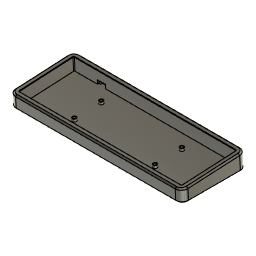
Quark MFR2 (Autodesk Fusion 360 design; units mm, degrees)
Autodesk Fusion 360 part; units mm, degrees
sketch "Sketch1" plane through (0, 0, 0) normal (0, 0, 1) x (1, 0, 0)
  line L0 (0, 0) -> (228.6, 0) construction
  line L1 (228.6, 0) -> (228.6, 76.2) construction
  line L2 (228.6, 76.2) -> (0, 76.2) construction
  line L3 (0, 76.2) -> (0, 0) construction
  line L4 (-0.5, -0.5) -> (229.1, -0.5)
  line L5 (229.1, -0.5) -> (229.1, 76.7)
  line L6 (229.1, 76.7) -> (-0.5, 76.7)
  line L7 (-0.5, 76.7) -> (-0.5, -0.5)
  line L8 (-7.5, 83.7) -> (-7.5, -7.5)
  line L9 (-7.5, -7.5) -> (236.1, -7.5)
  line L10 (236.1, -7.5) -> (236.1, 83.7)
  line L11 (236.1, 83.7) -> (-7.5, 83.7)
  dimension "d1" = 228.6
  dimension "d2" = 76.2
  dimension "d3" = 0.5
  dimension "d4" = 7.5
  constraint horizontal L0
  constraint vertical L1
  constraint horizontal L2
  constraint vertical L3
  constraint coincident L0.start L3.end
  measures "d1" distance of L0.start L0.end
  measures "d2" distance of L0.start L2.end
ref_plane "WorkPlane1" through (114.3, 38.1, -3.46) normal (0, 0, 1) x (1, 0, 0)
ref_plane "WorkPlane2" through (114.3, 38.1, 14.6) normal (0, 0, 1) x (1, 0, 0)
extrude "Extrude1" add sketch "Sketch1" along normal up to surface (14.6 mm away) and the other way up to surface (3.46 mm away)
sketch "Sketch3" plane through (236.1, 0, 0) normal (1, 0, 0) x (0, 1, 0)
  line L0 (83.7, 14.6) -> (-7.5, 14.6)
  line L1 (-7.5, 14.6) -> (-7.5, -3.46)
  line L2 (-7.5, -3.46) -> (83.7, -3.46)
  line L3 (83.7, -3.46) -> (83.7, 14.6)
  line L4 (-7.5, 14.6) -> (-7.5, -3.6755)
  line L5 (-7.5, -3.6755) -> (92.363, -8.9091)
  line L6 (-7.5, -3.6755) -> (92.5, -3.6755) construction
  dimension "d11" = 18.2755
  dimension "d12" = 100
  dimension "d13" = 3
  constraint coincident L0.end L1.start
  constraint perpendicular L0 L4
  constraint horizontal L6
  measures "d11" distance of L0.end L4.end
  measures "d12" distance of L4.end L5.end
  measures "d13" angle of L5 L6
ref_plane "WorkPlane3" through (236.1, 42.4315, -6.2923) normal (0, -0.052336, -0.99863) x (0, 0.99863, -0.052336)
sketch "Sketch5" plane through (0, 0, -3.46) normal (0, 0, -1) x (1, 0, 0)
  line L0 (229.1, -76.7) -> (-0.5, -76.7)
  line L1 (-0.5, -76.7) -> (-0.5, 0.5)
  line L2 (-0.5, 0.5) -> (229.1, 0.5)
  line L3 (229.1, 0.5) -> (229.1, -76.7)
  line L4 (-7.5, 7.5) -> (-7.5, -83.7)
  line L5 (-7.5, -83.7) -> (236.1, -83.7)
  line L6 (236.1, -83.7) -> (236.1, 7.5)
  line L7 (236.1, 7.5) -> (-7.5, 7.5)
  line L8 (-7.5, 7.5) -> (236.1, 7.5)
  line L9 (236.1, 7.5) -> (236.1, -83.7)
  line L10 (236.1, -83.7) -> (-7.5, -83.7)
  line L11 (-7.5, -83.7) -> (-7.5, 7.5)
  constraint horizontal L8
  constraint vertical L9
  constraint horizontal L10
  constraint vertical L11
  constraint coincident L5.end L6.start
  constraint coincident L4.start L7.end
extrude "Extrude2" add sketch "Sketch5" along normal up to surface contours L0 L1 L2 L3 | L4 L5 L6 L7 L8 L9 L10 L11 end surface through (236.1, 42.4315, -6.2923) normal (0, -0.052336, -0.99863) offset 0
fillet "Fillet1" radius 9 1 edges at (236.1, -7.5, 5.4623)
fillet "Fillet2" radius 9 1 edges at (236.1, 83.7, 3.0725)
fillet "Fillet3" radius 9 1 edges at (-7.5, 83.7, 3.0725)
fillet "Fillet4" radius 9 1 edges at (-7.5, -7.5, 5.4623)
fillet "Fillet5" radius 1 1 edges at (229.1, 76.7, 5.57)
fillet "Fillet6" radius 1 1 edges at (-0.5, 76.7, 5.57)
fillet "Fillet7" radius 1 1 edges at (229.1, -0.5, 5.57)
fillet "Fillet8" radius 1 1 edges at (-0.5, -0.5, 5.57)
chamfer "Chamfer1" distance 2 angle 45 8 edges at (-7.5, 38.1, 14.6) (-4.864, 81.064, 14.6) (114.3, 83.7, 14.6) (233.464, 81.064, 14.6) (236.1, 38.1, 14.6) (233.464, -4.864, 14.6) (114.3, -7.5, 14.6) (-4.864, -4.864, 14.6)
chamfer "Chamfer2" distance 2 angle 45 8 edges at (-7.5, 38.1, -6.0653) (-4.864, -4.864, -3.8136) (114.3, -7.5, -3.6755) (233.464, -4.864, -3.8136) (236.1, 38.1, -6.0653) (233.464, 81.064, -8.3169) (114.3, 83.7, -8.4551) (-4.864, 81.064, -8.3169)
chamfer "Chamfer3" distance 0.5 angle 45 4 edges at (114.3, 76.7, 14.6) (-0.5, 38.1, 14.6) (114.3, -0.5, 14.6) (229.1, 38.1, 14.6)
extrude "Extrude3" add 1 faces at (76.7, 52.6342, -6.827) along direction (0, 0.052336, 0.99863) blind 1
ref_plane "WorkPlane4" through (114.3, 38.1, 0) normal (0, 0, 1) x (1, 0, 0)
sketch "USB C Hole Internal" plane through (0, 76.7, 0) normal (0, -1, 0) x (1, 0, 0)
  line L0 (228.1, 14.1) -> (0.5, 14.1)
  line L1 (0.5, -3.46) -> (228.1, -3.46)
  line L2 (228.1, -3.46) -> (216.1938, -3.4777) construction
  line L3 (216.1938, -3.4777) -> (216.1883, 0.1823) construction
  line L4 (188.5829, -1.4386) -> (179.1329, -1.4526) construction
  line L5 (34.925, -3.46) -> (41.275, -3.46)
  line L6 (42.825, -1.91) -> (42.825, -1.35)
  line L7 (41.275, 0.2) -> (34.925, 0.2)
  line L8 (33.375, -1.35) -> (33.375, -1.91)
  arc A0 (34.925, 0.2) -> (33.375, -1.35) centre (34.925, -1.35) ccw
  arc A1 (42.825, -1.35) -> (41.275, 0.2) centre (41.275, -1.35) ccw
  arc A2 (41.275, -3.46) -> (42.825, -1.91) centre (41.275, -1.91) ccw
  arc A3 (33.375, -1.91) -> (34.925, -3.46) centre (34.925, -1.91) ccw
  line L9 (0.5, 14.1) -> (0.5, -3.46)
  line L10 (228.1, -3.46) -> (228.1, 14.1)
  line L11 (38.1, -3.46) -> (34.925, -3.46)
  dimension "d32" = 11.9062
  dimension "d33" = 3.66
  dimension "d35" = 9.45
  dimension "d36" = 1.55
  dimension "d82" = 38.1
  constraint coincident L1.end L2.start
  constraint perpendicular L2 L3
  constraint perpendicular L3 L4
  constraint horizontal L5
  constraint vertical L6
  constraint horizontal L7
  constraint vertical L8
  constraint tangent L8 A0
  constraint tangent L7 A0
  constraint tangent L7 A1
  constraint tangent L6 A1
  constraint equal A0 A1
  constraint tangent L5 A2
  constraint tangent L6 A2
  constraint equal A0 A2
  constraint tangent L5 A3
  constraint tangent L8 A3
  constraint equal A0 A3
  constraint midpoint L5 L11.start
  measures "d32" distance of L1.end L2.end
  measures "d33" distance of L2.end L3.end
  measures "d35" distance of L4.start L4.end
  measures "d36" radius of A0
  measures "d82" horizontal distance of L11.start origin
extrude "Extrude4" cut sketch "USB C Hole Internal" against normal through all contours L1 L5 L6 L7 L8 A0 A1 A2 A3 L11
sketch "Sketch8" plane through (0, 83.7, 0) normal (0, 1, 0) x (-1, 0, 0)
  line L0 (-41.275, 0.2) -> (-34.925, 0.2)
  arc A0 (-33.375, -1.35) -> (-34.925, 0.2) centre (-34.925, -1.35) ccw
  line L1 (-33.375, -1.35) -> (-33.375, -1.91)
  arc A1 (-34.925, -3.46) -> (-33.375, -1.91) centre (-34.925, -1.91) ccw
  line L2 (-34.925, -3.46) -> (-41.275, -3.46)
  arc A2 (-42.825, -1.91) -> (-41.275, -3.46) centre (-41.275, -1.91) ccw
  line L3 (-42.825, -1.91) -> (-42.825, -1.35)
  arc A3 (-41.275, 0.2) -> (-42.825, -1.35) centre (-41.275, -1.35) ccw
  line L4 (-227.1, -6.4551) -> (-1.5, -6.4551)
  line L5 (-1.5, -6.4551) -> (-1.5, 12.6)
  line L6 (-1.5, 12.6) -> (-227.1, 12.6)
  line L7 (-227.1, 12.6) -> (-227.1, -6.4551)
  line L8 (-33.375, -1.63) -> (-42.825, -1.63) construction
  line L9 (-38.1, 0.2) -> (-38.1, -3.46) construction
  line L10 (-41.275, 2.2669) -> (-34.925, 2.2669)
  line L11 (-31.125, -1.5331) -> (-31.125, -2.0931)
  line L12 (-34.925, -5.8931) -> (-41.275, -5.8931)
  line L13 (-45.075, -2.0931) -> (-45.075, -1.5331)
  arc A4 (-45.075, -2.0931) -> (-41.275, -5.8931) centre (-41.275, -2.0931) ccw
  arc A5 (-41.275, 2.2669) -> (-45.075, -1.5331) centre (-41.275, -1.5331) ccw
  arc A6 (-31.125, -1.5331) -> (-34.925, 2.2669) centre (-34.925, -1.5331) ccw
  arc A7 (-34.925, -5.8931) -> (-31.125, -2.0931) centre (-34.925, -2.0931) ccw
  line L14 (-45.075, -1.8131) -> (-31.125, -1.8131) construction
  line L15 (-38.1, 2.2669) -> (-38.1, -5.8931) construction
  line L16 (-38.1, -1.8131) -> (-45.075, -1.8131) construction
  line L17 (-38.1, -1.8131) -> (-38.1, 2.2669) construction
  line L18 (-42.825, -1.63) -> (-38.1, -1.63) construction
  dimension "d43" = 3.8
  dimension "d85" = 13.95
  dimension "d86" = 8.16
  dimension "d87" = 6.975
  constraint midpoint L1 L8.start
  constraint midpoint L3 L8.end
  constraint midpoint L0 L9.start
  constraint midpoint L2 L9.end
  constraint horizontal L10
  constraint vertical L11
  constraint horizontal L12
  constraint vertical L13
  constraint tangent L12 A4
  constraint tangent L13 A4
  constraint tangent L13 A5
  constraint tangent L10 A5
  constraint equal A4 A5
  constraint tangent L10 A6
  constraint tangent L11 A6
  constraint equal A4 A6
  constraint tangent L11 A7
  constraint tangent L12 A7
  constraint equal A4 A7
  constraint midpoint L13 L14.start
  constraint midpoint L11 L14.end
  constraint midpoint L10 L15.start
  constraint midpoint L12 L15.end
  constraint midpoint L14 L16.start
  constraint midpoint L8 L18.end
  measures "d43" radius of A4
  measures "d85" distance of L11 L13
  measures "d86" distance of L10 L12
  measures "d87" horizontal distance of L14.start L18.end
extrude "Extrude5" cut sketch "Sketch8" against normal blind 2.7025 contours L10 L11 L12 L13 A4 A5 A6 A7
chamfer "Chamfer4" distance 0.25 angle 45 8 edges at (43.962, 83.7, -4.7801) (45.075, 83.7, -1.8131) (43.962, 83.7, 1.154) (38.1, 83.7, 2.2669) (32.238, 83.7, 1.154) (31.125, 83.7, -1.8131) (32.238, 83.7, -4.7801) (38.1, 83.7, -5.8931)
sketch "Sketch9" plane through (0, 0, 0) normal (0, 0, 1) x (1, 0, 0)
  line L0 (0, 0) -> (228.6, 0) construction
  line L1 (228.6, 0) -> (228.6, 76.2) construction
  line L2 (228.6, 76.2) -> (0, 76.2) construction
  line L3 (0, 76.2) -> (0, 0) construction
  line L4 (228.6, 76.2) -> (228.6, 57.15) construction
  line L5 (228.6, 57.15) -> (193.1449, 57.15) construction
  circle A0 centre (171.3, 57.1) radius 2.75
  circle A1 centre (57.3, 57.1) radius 2.75
  circle A2 centre (57.3, 19.1) radius 2.75
  circle A3 centre (171.3, 19.1) radius 2.75
  dimension "d47" = 228.6
  dimension "d48" = 76.2
  dimension "d51" = 19.1
  dimension "d52" = 57.3
  dimension "d53" = 19.1
  dimension "d54" = 57.3
  dimension "d55" = 57.3
  dimension "d56" = 19.1
  dimension "d57" = 57.3
  dimension "d58" = 19.1
  dimension "d59" = 5.5
  constraint horizontal L0
  constraint vertical L1
  constraint horizontal L2
  constraint vertical L3
  constraint coincident L0.start L3.end
  constraint perpendicular L2 L4
  constraint perpendicular L1 L5
  constraint equal A0 A1
  constraint equal A0 A3
  constraint equal A1 A2
  measures "d47" distance of L0.start L0.end
  measures "d48" distance of L0.start L2.end
  measures "d51" distance of L2 A0.centre
  measures "d52" distance of L1 A0.centre
  measures "d53" distance of L0 A3.centre
  measures "d54" distance of L1 A3.centre
  measures "d55" distance of L3 A2.centre
  measures "d56" distance of L0 A2.centre
  measures "d57" distance of L3 A1.centre
  measures "d58" distance of L2 A1.centre
  measures "d59" diameter of A1
extrude "Extrude6" add sketch "Sketch9" against normal up to surface (3.46 mm away)
hole "Hole1" at (171.3, 19.1, 0) direction (0, 0, -1) diameter 3.2 depth 4 tip angle 180
hole "Hole2" at (171.3, 57.1, 0) direction (0, 0, -1) diameter 3.2 depth 4 tip angle 180
hole "Hole3" at (57.3, 19.1, 0) direction (0, 0, -1) diameter 3.2 depth 4 tip angle 180
hole "Hole4" at (57.3, 57.1, 0) direction (0, 0, -1) diameter 3.2 depth 4 tip angle 180
sketch "Sketch6" plane through (0, 0, -3.46) normal (0, 0, 1) x (-1, 0, 0)
  line L0 (0.5, -7.4953) -> (-229.1, -7.4953)
  line L1 (-229.1, -7.4953) -> (-229.1, -75.7)
  line L2 (-34.925, -76.7) -> (-0.5, -76.7)
  line L3 (0.5, -75.7) -> (0.5, -7.4953)
  circle A0 centre (-57.3, -19.1) radius 2.75
  circle A1 centre (-171.3, -57.1) radius 2.75
  circle A2 centre (-57.3, -57.1) radius 2.75
  circle A3 centre (-171.3, -19.1) radius 2.75
  line L4 (-34.925, -80.9975) -> (-34.925, -76.7)
  arc A4 (-0.5, -76.7) -> (0.5, -75.7) centre (-0.5, -75.7) ccw
  arc A5 (-229.1, -75.7) -> (-228.1, -76.7) centre (-228.1, -75.7) ccw
  line L5 (-228.1, -76.7) -> (-41.275, -76.7)
  line L6 (-41.275, -76.7) -> (-41.275, -80.9975)
  line L7 (-41.275, -80.9975) -> (-34.925, -80.9975)
sketch "Cutout for usb" plane through (0, 76.7, 0) normal (0, -1, 0) x (1, 0, 0)
  arc A0 (41.275, -3.46) -> (42.825, -1.91) centre (41.275, -1.91) ccw
  line L0 (41.275, -3.46) -> (228.1, -3.46)
  line L1 (228.1, -3.46) -> (228.1, 14.1)
  line L2 (228.1, 14.1) -> (0.5, 14.1)
  line L3 (0.5, 14.1) -> (0.5, -3.46)
  line L4 (0.5, -3.46) -> (34.925, -3.46)
  arc A1 (33.375, -1.91) -> (34.925, -3.46) centre (34.925, -1.91) ccw
  line L5 (33.375, -1.91) -> (33.375, -1.35)
  arc A2 (34.925, 0.2) -> (33.375, -1.35) centre (34.925, -1.35) ccw
  line L6 (34.925, 0.2) -> (41.275, 0.2)
  arc A3 (42.825, -1.35) -> (41.275, 0.2) centre (41.275, -1.35) ccw
  line L7 (42.825, -1.35) -> (42.825, -1.91)
  line L8 (32.375, -3.46) -> (43.825, -3.46)
  line L9 (43.825, -3.46) -> (43.825, 2.2)
  line L10 (43.825, 2.2) -> (32.375, 2.2)
  line L11 (32.375, 2.2) -> (32.375, -3.46)
  dimension "d88" = 1
  dimension "d89" = 1
  dimension "d90" = 2
  constraint horizontal L8
  constraint vertical L9
  constraint horizontal L10
  constraint vertical L11
  constraint coincident L4 L8.start
  measures "d88" distance of L5 L11
  measures "d89" distance of L7 L9
  measures "d90" distance of L6 L10
extrude "Extrude7" cut sketch "Cutout for usb" against normal blind 2 contours A0 L0 L4 A1 L5 A2 L6 A3 L7 L8 L9 L10 L11
move_body "Move1" bodies 1 to x (1, 0, 0) y (0, 0.99863, 0.052336) z (0, -0.052336, 0.99863) at (0, -0.098, 0.3902)
